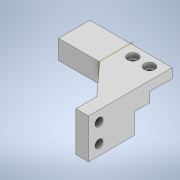
# Autodesk Inventor part: Non_compliant_plate2
Saved by Autodesk Inventor 2022 (Build 260153000, 153)
## iProperties
Created: 2021-08-01
Part Number: Non_compliant_plate2
Material: Generic
Document SubType Name: Modeling
Designer: exllu
Density: 1 g/cm^3
Appearance: Default
Author: exllu
Autodesk Inventor part; units mm, degrees
ref_plane "YZ Plane" through (0, 0, 0) normal (1, 0, 0) x (0, 1, 0)
ref_plane "XZ Plane" through (0, 0, 0) normal (0, 1, 0) x (-1, 0, 0)
ref_plane "XY Plane" through (0, 0, 0) normal (0, 0, 1) x (1, 0, 0)
sketch "Sketch1" plane through (0, 0, 0) normal (0, 1, 0) x (-1, 0, 0)
  line L0 (0, 0) -> (-19.65, 0)
  line L1 (-19.65, 0) -> (-19.65, -12)
  line L2 (-19.65, -12) -> (0, -12)
  line L3 (0, -12) -> (0, 0)
  line L4 (0, 0) -> (0, -6)
  line L5 (0, -6) -> (-5.825, -6)
  line L6 (-5.825, -6) -> (-13.825, -6)
  circle A0 centre (-5.825, -6) radius 1.05
  circle A1 centre (-13.825, -6) radius 1.05
  dimension "d0" = 19.65
  dimension "d1" = 12
  dimension "d2" = 6
  dimension "d3" = 5.825
  dimension "d4" = 8
  dimension "d5" = 2.1
  dimension "d6" = 2.1
  constraints: 14 end point, 4 coincident, 2 centre point, 2 horizontal, 2 parallel, 2 perpendicular, 1 midpoint
  measures "d0" distance of L2.end L1.end
  measures "d1" distance of L1.end L0.end
  measures "d2" distance of L0.start L4.end
  measures "d3" distance of L4.end L5.end
  measures "d4" distance of L5.end L6.end
  measures "d5" diameter of A0
  measures "d6" diameter of A1
extrude "Extrusion1" add sketch "Sketch1" along normal blind 4.5
sketch "Sketch2" plane through (0, 4.5, 0) normal (0, 1, 0) x (1, 0, 0)
  line L0 (0, 0) -> (19.65, 0) projected
  line L1 (0, 0) -> (0, 6)
  line L2 (0, 12) -> (0, 0) projected
  line L3 (0, 6) -> (5.825, 6)
  line L4 (5.825, 6) -> (13.825, 6)
  circle A0 centre (5.825, 6) radius 2.5
  circle A1 centre (13.825, 6) radius 2.5
  dimension "d9" = 5.825
  dimension "d10" = 8
  dimension "d11" = 5
  dimension "d12" = 5
  constraints: 6 end point, 2 centre point, 2 coincident, 1 midpoint, 1 perpendicular, 1 point on line
  measures "d9" distance of L1.end L3.end
  measures "d10" distance of L3.end L4.end
  measures "d11" diameter of A0
  measures "d12" diameter of A1
extrude "Extrusion2" cut sketch "Sketch2" against normal blind 2
sketch "Sketch3" plane through (0, 4.5, 0) normal (0, 1, 0) x (1, 0, 0)
  line L0 (19.65, 12) -> (0, 12) projected
  line L1 (0, 0) -> (3, 0)
  line L2 (3, 0) -> (3, 12)
  line L3 (3, 12) -> (0, 12)
  line L4 (0, 12) -> (0, 0)
  dimension "d15" = 3
  constraints: 8 end point, 2 parallel, 1 horizontal, 1 perpendicular, 1 point on line
  measures "d15" distance of L3.end L2.end
extrude "Extrusion3" add sketch "Sketch3" along normal blind 11.5
sketch "Sketch4" plane through (0, 16, 0) normal (0, 1, 0) x (1, 0, 0)
  line L0 (0, 0) -> (3, 0) projected
  line L1 (0, 0) -> (3, 0)
  line L2 (3, 0) -> (3, 1)
  line L3 (3, 0) -> (3, 12) projected
  line L4 (3, 1) -> (2, 1)
  line L5 (2, 1) -> (2, 11)
  line L6 (2, 11) -> (3, 11)
  line L7 (3, 1) -> (3, 11)
  dimension "d18" = 1
  dimension "d19" = 1
  dimension "d20" = 10
  constraints: 12 end point, 4 perpendicular, 2 point on line, 1 horizontal
  measures "d18" distance of L0.end L2.end
  measures "d19" distance of L2.end L4.end
  measures "d20" distance of L4.end L5.end
extrude "Extrusion4" cut sketch "Sketch4" against normal blind 11.5
sketch "Sketch6" plane through (0, 0, 0) normal (0, 0, 1) x (1, 0, 0)
  line L0 (0, 0) -> (19.65, 0) projected
  line L1 (0, 0) -> (5, 0)
  line L2 (5, 0) -> (5, 4.5)
  line L3 (3.325, 4.5) -> (8.325, 4.5) projected
  line L4 (19.65, 0) -> (19.65, 4.5) projected
  line L5 (19.65, 4.5) -> (19.65, 0)
  line L6 (19.65, 0) -> (5, 0)
  line L7 (5, 4.5) -> (19.65, 4.5)
  line L8 (19.65, 0) -> (5, 0)
  line L9 (19.65, 4.5) -> (19.65, -3.5)
  line L10 (5, 4.5) -> (-3, 4.5)
  line L11 (3, 4.5) -> (19.65, 4.5) projected
  line L12 (5, 4.5) -> (5, -3.5)
  line L13 (5, -3.5) -> (19.65, -3.5)
  dimension "d24" = 5
  dimension "d25" = 8
  dimension "d26" = 8
  dimension "d27" = 8
  constraints: 20 end point, 3 collinear, 3 point on line, 2 perpendicular, 1 horizontal, 1 vertical
  measures "d24" distance of L0.start L1.end
  measures "d25" distance of L4.end L9.end
  measures "d26" distance of L2.end L10.end
  measures "d27" distance of L2.end L12.end
extrude "Extrusion5" add sketch "Sketch6" along normal blind 2
sketch "Sketch7" plane through (0, 0, 2) normal (0, 0, 1) x (1, 0, 0)
  line L0 (5, 0) -> (5, -3.5) projected
  line L1 (5, -3.5) -> (11, -3.5)
  line L2 (11, -3.5) -> (11, 4.5)
  line L3 (11, 4.5) -> (5, 4.5)
  line L4 (5, 4.5) -> (5, -3.5)
  line L5 (5, -3.5) -> (19.65, -3.5) projected
  line L6 (5, -3.5) -> (11, -3.5)
  line L7 (11, -3.5) -> (11, -14.5)
  line L8 (11, -14.5) -> (5, -14.5)
  line L9 (5, -14.5) -> (5, -3.5)
  point P0 (0, 0)
  dimension "d30" = 6
  dimension "d31" = 8
  dimension "d32" = 6
  dimension "d33" = 11
  constraints: 16 end point, 4 parallel, 2 horizontal, 2 perpendicular
  measures "d30" distance of L3.end L2.end
  measures "d31" distance of L2.end L1.end
  measures "d32" distance of L7.end L8.end
  measures "d33" distance of L6.end L7.end
extrude "Extrusion6" add sketch "Sketch7" along normal blind 27
sketch "Sketch8" plane through (11, -14.5, 2) normal (1, 0, 0) x (0, 0, -1)
  line L0 (0, 11) -> (0, 0) projected
  line L1 (0, 0) -> (-27, 0)
  line L2 (0, 0) -> (-27, 0) projected
  line L3 (-27, 0) -> (-27, 5)
  line L4 (2, 19) -> (-27, 19) projected
  circle A0 centre (-27, 5) radius 2
  line L5 (0, 19) -> (-27, 19)
  line L6 (-27, 19) -> (-27, 14)
  circle A1 centre (-27, 14) radius 2
  line L7 (-27, 14) -> (-22, 14)
  line L8 (-27, 5) -> (-22, 5)
  circle A2 centre (-22, 14) radius 1.9305
  circle A3 centre (-22, 5) radius 1.9305
  point P0 (2, 14.5)
  point P1 (-25, 14)
  point P2 (-27, 16)
  point P3 (-25, 5)
  point P4 (-27, 3)
  dimension "d36" = 27
  dimension "d37" = 5
  dimension "d39" = 4
  dimension "d41" = 27
  dimension "d42" = 5
  dimension "d43" = 4
  dimension "d44" = 5
  dimension "d45" = 5
  dimension "d46" = 3.861
  dimension "d47" = 3.861
  constraints: 12 end point, 4 centre point, 4 coincident, 2 horizontal, 2 perpendicular, 2 point on line
  measures "d36" distance of L0.end L1.end
  measures "d37" distance of L1.end L3.end
  measures "d39" diameter of A0
  measures "d41" distance of L5.start L5.end
  measures "d42" distance of L5.end L6.end
  measures "d43" diameter of A1
  measures "d44" distance of L7.start L7.end
  measures "d45" distance of L8.start L8.end
  measures "d46" diameter of A2
  measures "d47" diameter of A3
sketch "Sketch10" plane through (11, -14.5, 2) normal (1, 0, 0) x (0, 0, -1)
  line L0 (0, 0) -> (-27, 0) projected
  line L1 (0, 0) -> (-5, 0)
  line L2 (-5, 0) -> (-5, 11)
  line L3 (-5, 11) -> (0, 11)
  line L4 (0, 11) -> (0, 0)
  point P0 (2, 14.5)
  point P1 (-5, 0)
  dimension "d52" = 5
  dimension "d53" = 11
  constraints: 8 end point, 2 parallel, 1 horizontal, 1 perpendicular
  measures "d52" distance of L2.end L3.end
  measures "d53" distance of L1.end L2.end
extrude "Extrusion9" cut sketch "Sketch10" against normal blind 20
sketch "Sketch11" plane through (11, -3.5, 2) normal (1, 0, 0) x (0, 0, -1)
  line L0 (-27, 8) -> (0, 8)
  line L1 (0, 8) -> (0, -11)
  line L2 (0, -11) -> (-27, -11)
  line L3 (-27, -11) -> (-27, 8)
  line L4 (-5, 0) -> (0, 0) projected
  line L5 (-5, 0) -> (0, 0)
  line L6 (0, 0) -> (0, -11)
  line L7 (0, -11) -> (-5, -11)
  line L8 (-5, -11) -> (-5, 0)
  point P0 (2, 3.5)
  dimension "d56" = 27
  dimension "d57" = 19
  constraints: 16 end point, 4 parallel, 2 horizontal, 2 perpendicular
  measures "d56" distance of L1.end L2.end
  measures "d57" distance of L0.end L1.end
extrude "Extrusion10" add sketch "Sketch11" along normal blind 16 contours L0 L1 L4 L8 L2 L3
sketch "Sketch13" plane through (5, -3.5, 0) normal (-1, 0, 0) x (0, 0, 1)
  line L0 (0, 3.5) -> (0, 8) projected
  line L1 (0, 8) -> (30.196, 8)
  line L2 (30.196, 8) -> (30.196, -11.8084)
  line L3 (30.196, -11.8084) -> (0, -11.8084)
  line L4 (0, -11.8084) -> (0, 8)
  constraints: 8 end point, 2 parallel, 1 horizontal, 1 perpendicular
extrude "Extrusion12" cut sketch "Sketch13" against normal blind 12.5
extrude "Extrusion13" cut sketch "Sketch8" along normal blind 30 contours A2 | A3
sketch "Sketch14" plane through (0, 0, -12) normal (-1, 0, 0) x (0, 0, 1)
  line L0 (12, 4.5) -> (12, 16) projected
  line L1 (12, 4.5) -> (16, 4.5)
  line L2 (14, 4.5) -> (41, 4.5) projected
  line L3 (12, 4.5) -> (12, 0) projected
  line L4 (16, 4.5) -> (12, 4.5)
  line L5 (12, 4.5) -> (12, 0)
  line L6 (12, 0) -> (16, 0)
  line L7 (16, 0) -> (16, 4.5)
  line L8 (16, 0) -> (12, 0)
  line L9 (12, 0) -> (12, -3.5)
  line L10 (12, -3.5) -> (16, -3.5)
  line L11 (16, -3.5) -> (16, 0)
  dimension "d68" = 4
  dimension "d69" = 3.5
  constraints: 18 end point, 4 parallel, 2 horizontal, 2 perpendicular, 2 point on line
  measures "d68" distance of L0.start L1.end
  measures "d69" distance of L9.end L8.end
extrude "Extrusion14" add sketch "Sketch14" against normal blind 27
sketch "Sketch15" plane through (27, -3.5, 2) normal (1, 0, 0) x (0, 0, -1)
  line L0 (-27.7224, 9.1153) -> (2, 9.1153)
  line L1 (2, 9.1153) -> (2, -11.9629)
  line L2 (2, -11.9629) -> (-27.7224, -11.9629)
  line L3 (-27.7224, -11.9629) -> (-27.7224, 9.1153)
  point P0 (2, 3.5)
  constraints: 8 end point, 2 parallel, 1 horizontal, 1 perpendicular
extrude "Extrusion15" cut sketch "Sketch15" against normal blind 3.5
sketch "Sketch16" plane through (0, 0, 0) normal (0, 0, -1) x (-1, 0, 0)
  line L0 (-23.5, 4.5) -> (-23.5, -3.5) projected
  line L1 (-19.65, 0) -> (0, 0) projected
  line L2 (-23.5, 4.5) -> (-19.65, 4.5)
  line L3 (-19.65, 4.5) -> (-19.65, 0)
  line L4 (-19.65, 0) -> (-23.5, 0)
  line L5 (-23.5, 0) -> (-23.5, 4.5)
  line L6 (0, -3.5) -> (-23.5, -3.5) projected
  line L7 (-23.5, -3.5) -> (0, -3.5)
  line L8 (0, -3.5) -> (0, 0)
  line L9 (0, 0) -> (-23.5, 0)
  line L10 (-23.5, 0) -> (-23.5, -3.5)
  constraints: 16 end point, 4 parallel, 2 horizontal, 2 perpendicular
extrude "Extrusion16" cut sketch "Sketch16" against normal blind 0.25
chamfer "Chamfer2" distance 11.5 angle 22.5 1 edges at (3, 4.5, -0.5) measured on face at (3, 8.3333, -0.6667)
chamfer "Chamfer3" distance 11.5 angle 22.5 1 edges at (3, 4.5, -11.5) measured on face at (3, 8.3333, -11.3333)
sketch "Sketch17" plane through (17.5, -3.5, 0) normal (-1, 0, 0) x (0, 0, 1)
  line L0 (4, 8) -> (0, 8) projected
  line L1 (4, 8) -> (29, 8) projected
  line L2 (4, 8) -> (29, 8)
  line L3 (29, -11) -> (7, -11) projected
  line L4 (29, 8) -> (29, -11)
  line L5 (29, -11) -> (7, -11)
  line L6 (7, -11) -> (7, 0) projected
  line L7 (7, -11) -> (7, 0)
  line L8 (7, 0) -> (4, 0) projected
  line L9 (7, 0) -> (4, 0)
  line L10 (4, 0) -> (4, 8) projected
  line L11 (4, 0) -> (4, 8)
  circle A0 centre (24, 3) radius 1.9305 projected
  circle A1 centre (24, 3) radius 1.9305
  circle A2 centre (24, -6) radius 1.9305 projected
  circle A3 centre (24, -6) radius 1.9305
  point P0 (0, 3.5)
  constraints: 12 end point, 4 collinear, 2 centre point, 2 coincident, 2 perpendicular
extrude "Extrusion17" add sketch "Sketch17" along normal blind 7.75
sketch "Sketch19" plane through (19.65, 0, -12) normal (1, 0, 0) x (0, 0, -1)
  line L0 (3.0047, 17.6779) -> (-43.6886, 17.6779)
  line L1 (-43.6886, 17.6779) -> (-43.6886, -24.1526)
  line L2 (-43.6886, -24.1526) -> (3.0047, -24.1526)
  line L3 (3.0047, -24.1526) -> (3.0047, 17.6779)
  point P0 (-12, 0)
  constraints: 8 end point, 2 parallel, 1 horizontal, 1 perpendicular
extrude "Extrusion18" cut sketch "Sketch19" along normal blind 7.75
sketch "Sketch20" plane through (19.65, 0, -12) normal (1, 0, 0) x (0, 0, -1)
  line L0 (-16, -3.5) -> (-19, -3.5) projected
  line L1 (-41, 4.5) -> (-16, 4.5) projected
  line L2 (-16, -3.5) -> (-41, -3.5)
  line L3 (-41, -3.5) -> (-41, 4.5)
  line L4 (-41, 4.5) -> (-16, 4.5)
  line L5 (-16, 4.5) -> (-16, -3.5)
  line L6 (-19, -3.5) -> (-19, -14.5) projected
  line L7 (0, 4.5) -> (-41, 4.5) projected
  line L8 (-19, -14.5) -> (-41, -14.5)
  line L9 (-41, -14.5) -> (-41, 4.5)
  line L10 (-41, 4.5) -> (-19, 4.5)
  line L11 (-19, 4.5) -> (-19, -14.5)
  point P0 (-12, 0)
  constraints: 16 end point, 4 parallel, 2 horizontal, 2 perpendicular
extrude "Extrusion19" cut sketch "Sketch20" against normal blind 3.4
sketch "Sketch22" plane through (9.75, -3.5, 0) normal (-1, 0, 0) x (0, 0, 1)
  line L0 (29, 8) -> (4, 8) projected
  line L1 (29, -11) -> (29, 8) projected
  line L2 (4, 8) -> (29, 8)
  line L3 (29, 8) -> (29, -11)
  line L4 (29, -11) -> (4, -11)
  line L5 (4, -11) -> (4, 8)
  point P0 (0, 3.5)
  constraints: 8 end point, 2 parallel, 1 horizontal, 1 perpendicular
extrude "Extrusion21" cut sketch "Sketch22" against normal blind 0.5
chamfer "Chamfer6" distance 6 angle 45 1 edges at (10.25, 0.5, 4)
sketch "Sketch23" plane through (10.25, -3.5, 0) normal (-1, 0, 0) x (0, 0, 1)
  line L0 (0.25, 0) -> (4, 0) projected
  line L1 (29, -11) -> (0.25, -11)
  line L2 (0.25, -11) -> (0.25, 0)
  line L3 (0.25, 0) -> (29, 0)
  line L4 (29, 0) -> (29, -11)
  point P0 (0, 3.5)
  constraints: 8 end point, 2 parallel, 1 horizontal, 1 perpendicular
extrude "Extrusion22" cut sketch "Sketch23" along normal blind 6
chamfer "Chamfer7" distance 3 angle 45 1 edges at (10.25, -9, 7)
sketch "Sketch24" plane through (2, 4.5, -11) normal (0, 0, 1) x (1, 0, 0)
  line L0 (0, 11.5) -> (0, 0) projected
  line L1 (0, 11.5) -> (1, 11.5) projected
  line L2 (0, 11.5) -> (1, 11.5)
  line L3 (1, 11.5) -> (5.7635, 0) projected
  line L4 (1, 11.5) -> (5.7635, 0)
  line L5 (5.7635, 0) -> (0, 0)
  line L6 (0, 0) -> (0, 11.5)
  point P0 (-2, -4.5)
  constraints: 8 end point, 2 collinear, 1 parallel, 1 perpendicular
extrude "Extrusion23" add sketch "Sketch24" along normal blind 1
sketch "Sketch25" plane through (19.65, 0, -12) normal (0, 0, -1) x (-1, 0, 0)
  line L0 (11.8865, 4.5) -> (16.65, 16) projected
  line L1 (11.8865, 4.5) -> (21.5602, 4.5)
  line L2 (21.5602, 4.5) -> (21.5602, 16.6717)
  line L3 (21.5602, 16.6717) -> (11.8865, 16.6717)
  line L4 (11.8865, 16.6717) -> (11.8865, 4.5)
  point P0 (19.65, 0)
  constraints: 8 end point, 2 parallel, 1 horizontal, 1 perpendicular
extrude "Extrusion24" cut sketch "Sketch25" against normal blind 1
sketch "Sketch26" plane through (19.65, 0, -12) normal (0, 0, -1) x (-1, 0, 0)
  line L0 (23.0227, -5.5896) -> (-3.5888, -5.5896)
  line L1 (-3.5888, -5.5896) -> (-3.5888, 1.5983)
  line L2 (23.0227, 1.5983) -> (23.0227, -5.5896)
  line L3 (23.0227, -5.5896) -> (-3.178, -5.5896)
  line L4 (-3.178, -5.5896) -> (-3.178, 11.4907)
  line L5 (-3.178, 11.4907) -> (23.0227, 11.4907)
  line L6 (23.0227, 11.4907) -> (23.0227, -5.5896)
  point P0 (19.65, 0)
  constraints: 14 end point, 3 parallel, 2 horizontal, 2 perpendicular
extrude "Extrusion25" cut sketch "Sketch26" against normal blind 1
sketch "Sketch27" plane through (0, 0, 0.25) normal (0, 0, -1) x (-1, 0, 0)
  line L0 (-19.65, 0) -> (0, 0) projected
  line L1 (-19.65, -3.5) -> (-16.25, -3.5) projected
  line L2 (0, 0) -> (-19.65, 0)
  line L3 (-19.65, 0) -> (-19.65, -3.5)
  line L4 (-19.65, -3.5) -> (0, -3.5)
  line L5 (0, -3.5) -> (0, 0)
  constraints: 8 end point, 2 parallel, 1 horizontal, 1 perpendicular
extrude "Extrusion26" add sketch "Sketch27" along normal blind 0.25
sketch "Sketch28" plane through (0, 0, 0) normal (0, 0, -1) x (-1, 0, 0)
  line L0 (0, 0) -> (-19.65, 0) projected
  line L1 (-19.65, 0) -> (-19.65, -3.5) projected
  line L2 (0, 0) -> (-19.65, 0)
  line L3 (-19.65, 0) -> (-19.65, -3.5)
  line L4 (-19.65, -3.5) -> (0, -3.5)
  line L5 (0, -3.5) -> (0, 0)
  constraints: 8 end point, 2 parallel, 1 horizontal, 1 perpendicular
extrude "Extrusion27" add sketch "Sketch28" along normal blind 0.25
sketch "Sketch29" plane through (16.25, 0, -12) normal (1, 0, 0) x (0, 0, -1)
  line L0 (-16, -3.5) -> (-16, 4.5) projected
  line L1 (-19, -14.5) -> (-41, -14.5) projected
  line L2 (-16, 4.5) -> (-41, 4.5)
  line L3 (-41, 4.5) -> (-41, -14.5)
  line L4 (-41, -14.5) -> (-16, -14.5)
  line L5 (-16, -14.5) -> (-16, 4.5)
  line L6 (-19, -3.5) -> (-19, -14.5) projected
  line L7 (-19, -3.5) -> (-16, -3.5)
  line L8 (-16, -3.5) -> (-16, -14.5)
  line L9 (-16, -14.5) -> (-19, -14.5)
  line L10 (-19, -14.5) -> (-19, -3.5)
  circle A0 centre (-36, -0.5) radius 1.9305 projected
  circle A1 centre (-36, -0.5) radius 1.9305
  circle A2 centre (-36, -9.5) radius 1.9305 projected
  circle A3 centre (-36, -9.5) radius 1.9305
  point P0 (-12, 0)
  constraints: 16 end point, 4 parallel, 2 centre point, 2 coincident, 2 horizontal, 2 perpendicular
extrude "Extrusion28" add sketch "Sketch29" along normal blind 3.4 contours L7 L6 L1 L3 L2 L0
sketch "Sketch30" plane through (0, -3.5, 4) normal (0, -1, 0) x (1, 0, 0)
  line L0 (19.65, 3) -> (19.65, -4.25) projected
  line L1 (0, -15) -> (0, -4.25) projected
  line L2 (0, 3) -> (0, -4.25)
  line L3 (0, -4.25) -> (19.65, -4.25)
  line L4 (19.65, -4.25) -> (19.65, 3)
  line L5 (10.25, 6) -> (13.25, 3) projected
  line L6 (13.25, 3) -> (10.25, 6)
  line L7 (10.25, 6) -> (7.25, 3)
  line L8 (10.25, 6) -> (4.25, 0) projected
  line L9 (0, 0) -> (4.25, 0) projected
  line L10 (7.25, 3) -> (4.25, 0)
  line L11 (19.65, 3) -> (13.25, 3)
  line L12 (7.25, 3) -> (0, 3)
  point P0 (0, -4)
  constraints: 17 end point, 3 parallel, 2 collinear, 2 horizontal, 2 perpendicular, 1 midpoint
extrude "Extrusion29" add sketch "Sketch30" along normal blind 1.2 contours L0 L3 L2 L9 L8 L7 L5 L11
sketch "Sketch31" plane through (10.25, -3.5, 0) normal (-1, 0, 0) x (0, 0, 1)
  line L0 (29, 8) -> (29, -11) projected
  line L1 (29, -11) -> (10, -11) projected
  line L2 (29, 8) -> (19, 8)
  line L3 (19, 8) -> (19, -11)
  line L4 (19, -11) -> (29, -11)
  line L5 (29, -11) -> (29, 8)
  point P0 (0, 3.5)
  dimension "d126" = 10
  constraints: 8 end point, 2 parallel, 1 horizontal, 1 perpendicular, 1 point on line
  measures "d126" distance of L4.end L3.end
extrude "Extrusion30" cut sketch "Sketch31" against normal blind 3.4
sketch "Sketch32" plane through (0, 4.5, 0) normal (0, 1, 0) x (1, 0, 0)
  line L0 (13.65, -19) -> (10.25, -19) projected
  line L1 (10.25, -19) -> (10.25, -10) projected
  line L2 (13.65, -19) -> (10.25, -10)
  line L3 (10.25, -10) -> (7.9334, -20.7068)
  line L4 (7.9334, -20.7068) -> (13.65, -19)
  point P0 (0, 0)
  constraints: 6 end point
extrude "Extrusion31" cut sketch "Sketch32" against normal blind 20 contours L0 L1 L2
sketch "Sketch38" plane through (0, -4.7, 4) normal (0, -1, 0) x (1, 0, 0)
  line L0 (13.65, 15) -> (13.65, 3)
  line L1 (13.25, 3) -> (19.65, 3) projected
  line L2 (13.65, 3) -> (6.6933, 3)
  line L3 (10.25, 6) -> (13.65, 15) projected
  line L4 (6.6933, 3) -> (13.65, 15)
  point P0 (0, -4)
  constraints: 6 end point, 1 horizontal, 1 point on line, 1 vertical
extrude "Extrusion35" cut sketch "Sketch38" along normal blind 20
sketch "Sketch39" plane through (0, -4.7, 4) normal (0, -1, 0) x (1, 0, 0)
  line L0 (10.25, 6) -> (13.65, 15) projected
  line L1 (10.25, 6) -> (10.9568, 7.8709)
  line L2 (10.9568, 7.8709) -> (13.65, 7.8709)
  line L3 (13.65, 3) -> (13.65, 15) projected
  line L4 (13.65, 3) -> (10.9568, 3)
  line L5 (10.9568, 3) -> (10.9568, 7.8709)
  line L6 (10.9568, 7.8709) -> (13.65, 7.8709)
  line L7 (13.65, 7.8709) -> (13.65, 3)
  point P0 (0, -4)
  dimension "d150" = 2
  constraints: 12 end point, 2 horizontal, 2 parallel, 2 point on line, 1 perpendicular
  measures "d150" distance of L0.start L1.end
extrude "Extrusion36" add sketch "Sketch39" along normal blind 9.8 contours L2 L3 L4 L5
sketch "Sketch40" plane through (0, -4.7, 4) normal (0, -1, 0) x (1, 0, 0)
  line L0 (10.25, 6) -> (10.9568, 7.8709) projected
  line L1 (13.65, 25) -> (13.65, 7.8709) projected
  line L2 (10.9568, 7.8709) -> (13.65, 7.8709)
  line L3 (13.65, 15) -> (13.65, 25) projected
  line L4 (13.65, 7.8709) -> (13.65, 15)
  line L5 (10.9568, 7.8709) -> (13.65, 15) projected
  line L6 (13.65, 15) -> (10.9568, 7.8709)
  point P0 (0, -4)
  constraints: 6 end point, 1 collinear, 1 horizontal, 1 perpendicular
extrude "Extrusion37" add sketch "Sketch40" along normal blind 9.8
sketch "Sketch42" plane through (0, -4.7, 4) normal (0, -1, 0) x (1, 0, 0)
  line L0 (4.25, 0) -> (0, 0) projected
  line L1 (10.25, 6) -> (13.65, 15) projected
  line L2 (0, 0) -> (13.65, 15)
  line L3 (13.65, 15) -> (13.65, 4.5)
  line L4 (13.65, 4.5) -> (6.0124, 0)
  line L5 (0, 0) -> (4.25, 0) projected
  line L6 (6.0124, 0) -> (0, 0)
  point P0 (0, -4)
  constraints: 8 end point, 1 collinear, 1 vertical
extrude "Extrusion38" add sketch "Sketch42" against normal blind 9.2
sketch "Sketch45" plane through (19.65, -14.5, 7) normal (0, -1, 0) x (1, 0, 0)
  line L0 (-6, 12) -> (-19.65, -3) projected
  line L1 (-6, 12) -> (-11.8966, 12)
  line L2 (-11.8966, 12) -> (-11.8966, -1.0489)
  line L3 (-11.8966, -1.0489) -> (-6, -1.0489)
  line L4 (-6, -1.0489) -> (-6, 12)
  point P0 (-19.65, -7)
  point P1 (-11.8966, 5.5202)
  constraints: 8 end point, 2 parallel, 1 horizontal, 1 perpendicular
extrude "Extrusion40" cut sketch "Sketch45" against normal blind 9.8 contours L4 L3 L2 L0
chamfer "Chamfer12" distance 5.5 angle 47.7 1 edges at (13.65, -9.6, 7) measured on face at (17.65, -11.2333, 7)
fillet "Fillet6" radius 4 1 edges at (13.65, -9.6, 13.0444)
sketch "Sketch46" plane through (0, 4.5, 0) normal (-1, 0, 0) x (0, 0, 1)
  line L0 (-11, 0) -> (29, 0) projected
  line L1 (-11, 0) -> (2.4776, 0)
  line L2 (2.4776, 0) -> (2.4776, 14.1747)
  line L3 (2.4776, 14.1747) -> (-11, 14.1747)
  line L4 (-11, 14.1747) -> (-11, 0)
  point P0 (0, -4.5)
  point P1 (2.4776, 0)
  constraints: 8 end point, 2 parallel, 1 horizontal, 1 perpendicular
extrude "Extrusion41" cut sketch "Sketch46" against normal blind 40
sketch "Sketch47" plane through (0, 0, -11) normal (-1, 0, 0) x (0, 0, 1)
  line L0 (10.75, 0) -> (10.75, -4.7) projected
  line L1 (0, 0) -> (10.75, 0) projected
  line L2 (10.75, -4.7) -> (0, -4.7)
  line L3 (0, -4.7) -> (0, 0)
  line L4 (0, 0) -> (10.75, 0)
  line L5 (10.75, 0) -> (10.75, -4.7)
  line L6 (0, 0) -> (0, 4.5) projected
  line L7 (15, -4.7) -> (15, 4.5) projected
  line L8 (0, 4.5) -> (15, 4.5)
  line L9 (15, 4.5) -> (15, -4.7)
  line L10 (15, -4.7) -> (0, -4.7)
  line L11 (0, -4.7) -> (0, 4.5)
  point P0 (11, 0)
  point P1 (15, 4.5)
  constraints: 16 end point, 4 parallel, 2 horizontal, 2 perpendicular
ref_plane "Work Plane1" through (0, 0, -11) normal (-1, 0, 0) x (0, 0, 1)
extrude "Extrusion42" add sketch "Sketch47" along normal blind 19.65 contours L1 L6 L8 L7 L10 L0
body "Solid1"
